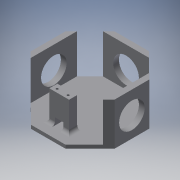
# Autodesk Inventor part: Main_assy_base
Saved by Autodesk Inventor 2017 (Build 210142000, 142)
## iProperties
Created: 2018-02-28
Part Number: Main_assy_base
Material: Generic
Document SubType Name: Modeling
Designer: Mitch
Density: 1 g/cm^3
Appearance: Default
Author: Mitch
Autodesk Inventor part; units mm, degrees
ref_plane "YZ Plane" through (0, 0, 0) normal (1, 0, 0) x (0, 1, 0)
ref_plane "XZ Plane" through (0, 0, 0) normal (0, 1, 0) x (-1, 0, 0)
ref_plane "XY Plane" through (0, 0, 0) normal (0, 0, 1) x (1, 0, 0)
sketch "Sketch1" plane through (0, 0, 0) normal (0, 1, 0) x (-1, 0, 0)
  line L0 (15.8302, -38.0798) -> (-15.7328, -38.1201)
  line L1 (-15.7328, -38.1201) -> (-38.0798, -15.8302)
  line L2 (-38.0798, -15.8302) -> (-38.1201, 15.7328)
  line L3 (-38.1201, 15.7328) -> (-15.8302, 38.0798)
  line L4 (-15.8302, 38.0798) -> (15.7328, 38.1201)
  line L5 (15.7328, 38.1201) -> (38.0798, 15.8302)
  line L6 (38.0798, 15.8302) -> (38.1201, -15.7328)
  line L7 (38.1201, -15.7328) -> (15.8302, -38.0798)
  point P0 (0, 0)
  point P1 (0, 0)
  dimension "d0" = 76.2
  constraints: 16 end point, 1 coincident, 17 other
  measures "d0" distance between parallel lines of L0 L4
extrude "Extrusion1" add sketch "Sketch1" along normal blind 3.175
sketch "Sketch3" plane through (0, 3.175, 0) normal (0, 1, 0) x (1, 0, 0)
  line L0 (38.1201, -15.7328) -> (38.0798, 15.8302) projected
  line L1 (-38.1201, 15.7328) -> (-38.0798, -15.8302) projected
  line L2 (32.9198, -20.9465) -> (32.8661, 21.0306)
  line L3 (-32.9198, 20.9465) -> (-32.8661, -21.0306)
  line L4 (-38.1201, 15.7328) -> (-38.0798, -15.8302) projected
  line L5 (38.1201, -15.7328) -> (38.0798, 15.8302) projected
  line L6 (38.1201, -15.7328) -> (32.9198, -20.9465)
  line L7 (38.0798, 15.8302) -> (38.1201, -15.7328) projected
  line L8 (38.1201, -15.7328) -> (38.0798, 15.8302)
  line L9 (38.0798, 15.8302) -> (32.8661, 21.0306)
  line L10 (-32.9198, 20.9465) -> (-38.1201, 15.7328)
  line L11 (-38.1201, 15.7328) -> (-38.0798, -15.8302)
  line L12 (-38.0798, -15.8302) -> (-38.1201, 15.7328) projected
  line L13 (-38.0798, -15.8302) -> (-32.8661, -21.0306)
  line L14 (-38.0798, -15.8302) -> (-15.7328, -38.1201) projected
  line L15 (15.8302, -38.0798) -> (38.1201, -15.7328) projected
  line L16 (38.0798, 15.8302) -> (15.7328, 38.1201) projected
  line L17 (38.1201, -15.7328) -> (32.9198, -20.9465)
  line L18 (38.0798, 15.8302) -> (32.8661, 21.0306)
  line L19 (15.7328, 38.1201) -> (38.0798, 15.8302) projected
  line L20 (38.1201, -15.7328) -> (38.0798, 15.8302)
  point P0 (0, 0)
  dimension "d5" = 5.207
  dimension "d6" = 5.207
  constraints: 22 end point, 4 collinear, 2 parallel, 1 perpendicular
  measures "d5" distance between parallel lines of L0 L2
  measures "d6" distance between parallel lines of L1 L3
extrude "Extrusion2" add sketch "Sketch3" along normal blind 35.56
sketch "Sketch5" plane through (38.0798, 0, -15.8302) normal (1, 0, -0.0013) x (-0.0013, 0, -1)
  circle A0 centre (-15.7815, 18.415) radius 11.43 projected
  circle A1 centre (-15.7815, 18.415) radius 11.684
  point P0 (-15.7815, 0)
  dimension "d9" = 0.254
  constraints: 1 centre point
  measures "d9" radial gap between concentric circles of A0 A1
extrude "Extrusion3" cut sketch "Sketch5" against normal blind 26.416 contours A0 | A1
sketch "Sketch6" plane through (-38.0798, 0, 15.8302) normal (-1, 0, 0.0013) x (0.0013, 0, 1)
  circle A0 centre (-15.7815, 18.415) radius 11.43 projected
  circle A1 centre (-15.7815, 18.415) radius 11.684
  point P0 (-15.7815, 0)
  dimension "d12" = 0.254
  constraints: 1 centre point
  measures "d12" radial gap between concentric circles of A0 A1
extrude "Extrusion4" cut sketch "Sketch6" against normal blind 26.416 contours A0 | A1
sketch "Sketch7" plane through (0, 3.175, 0) normal (0, 1, 0) x (1, 0, 0)
  line L0 (15.7328, 38.1201) -> (-15.8302, 38.0798) projected
  line L1 (20.9465, 32.9198) -> (-21.0306, 32.8661)
  line L2 (-15.8302, 38.0798) -> (-32.9198, 20.9465) projected
  line L3 (32.8661, 21.0306) -> (15.7328, 38.1201) projected
  line L4 (-38.1201, 15.7328) -> (-15.8302, 38.0798) projected
  line L5 (-21.0306, 32.8661) -> (-15.8302, 38.0798)
  line L6 (-15.8302, 38.0798) -> (15.7328, 38.1201)
  line L7 (20.9465, 32.9198) -> (15.7328, 38.1201)
  point P0 (0, 0)
  dimension "d15" = 5.207
  constraints: 8 end point, 4 point on line, 2 collinear, 1 parallel
  measures "d15" distance between parallel lines of L0 L1
extrude "Extrusion5" add sketch "Sketch7" along normal blind 35.56
sketch "Sketch8" plane through (-15.8302, 0, -38.0798) normal (-0.0013, 0, -1) x (-1, 0, 0.0013)
  circle A0 centre (-15.7815, 18.415) radius 11.43 projected
  circle A1 centre (-15.7815, 18.415) radius 11.684
  point P0 (-15.7815, 0)
  dimension "d18" = 0.254
  constraints: 1 centre point
  measures "d18" radial gap between concentric circles of A0 A1
extrude "Extrusion6" cut sketch "Sketch8" against normal blind 26.416 contours A0 | A1
sketch "Sketch9" plane through (0, 3.175, 0) normal (0, 1, 0) x (1, 0, 0)
  line L0 (-9.3728, -20.3542) -> (-9.3647, -26.7042) projected
  line L1 (8.6353, -26.6812) -> (8.6272, -20.3312) projected
  line L2 (-8.3634, -27.7029) -> (7.6366, -27.6825) projected
  line L3 (-9.3728, -20.3542) -> (8.6366, -20.3542)
  line L4 (8.6366, -20.3542) -> (8.6366, -27.6812)
  line L5 (8.6366, -27.6812) -> (-9.3728, -27.6812)
  line L6 (-9.3728, -27.6812) -> (-9.3728, -20.3542)
  point P0 (0, 0)
  constraints: 8 end point, 2 parallel, 1 horizontal, 1 perpendicular
extrude "Extrusion7" add sketch "Sketch9" along normal blind 26.67
sketch "Sketch10" plane through (0, 29.845, 0) normal (0, 1, 0) x (1, 0, 0)
  arc A0 (-5.3692, -23.1491) -> (-5.3658, -25.8491) centre (-5.3675, -24.4991) ccw projected
  arc A1 (-5.3658, -25.8491) -> (-5.3692, -23.1491) centre (-5.3675, -24.4991) ccw projected
  arc A2 (4.6308, -23.1363) -> (4.6342, -25.8363) centre (4.6325, -24.4863) ccw projected
  arc A3 (4.6342, -25.8363) -> (4.6308, -23.1363) centre (4.6325, -24.4863) ccw projected
  circle A4 centre (-5.3675, -24.4991) radius 1.016
  circle A5 centre (4.6325, -24.4863) radius 1.016
  point P0 (0, 0)
  dimension "d24" = 1.35
  dimension "d25" = 2.032
  dimension "d26" = 2.032
  constraints: 2 centre point, 2 coincident
  measures "d24" radius of A1
  measures "d25" diameter of A4
  measures "d26" diameter of A5
extrude "Extrusion8" cut sketch "Sketch10" against normal blind 12.7 contours A4 | A5
sketch "Sketch11" plane through (-9.3728, 3.175, 27.6812) normal (0, 0, 1) x (1, 0, 0)
  line L0 (18.0094, 0) -> (0, 0) projected
  line L1 (5.1947, 6.35) -> (12.8147, 6.35)
  line L2 (12.8147, 6.35) -> (12.8147, 0)
  line L3 (12.8147, 0) -> (5.1947, 0)
  line L4 (5.1947, 0) -> (5.1947, 6.35)
  line L5 (18.0094, 0) -> (18.0094, 26.67) projected
  point P0 (9.3728, -3.175)
  dimension "d31" = 5.1947
  dimension "d32" = 7.62
  dimension "d33" = 6.35
  dimension "d36" = 0
  constraints: 8 end point, 2 parallel, 1 horizontal, 1 perpendicular
  measures "d31" distance between parallel lines of L5 L2
  measures "d32" distance of L1.start L1.end
  measures "d33" distance between parallel lines of L0 L1
  measures "d36" distance between parallel lines of L0 L3
extrude "Extrusion9" cut sketch "Sketch11" against normal blind 12.7
fillet "Fillet2" radius 3.175 4 edges at (-6.7754, 3.175, 27.6812) (-9.3728, 3.175, 24.0177) (6.0392, 3.175, 27.6812) (8.6366, 3.175, 24.0177)
body "Solid1"
